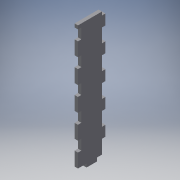
# Autodesk Inventor part: Part2
Saved by Autodesk Inventor 2018 (Build 220112000, 112)
## iProperties
Created: 2018-05-22
Part Number: Part2
Material: Generic
Document SubType Name: Modeling
Designer: Administrator
Density: 1 g/cm^3
Appearance: Default
Author: Administrator
Autodesk Inventor part; units mm, degrees
ref_plane "YZ Plane" through (0, 0, 0) normal (1, 0, 0) x (0, 1, 0)
ref_plane "XZ Plane" through (0, 0, 0) normal (0, 1, 0) x (-1, 0, 0)
ref_plane "XY Plane" through (0, 0, 0) normal (0, 0, 1) x (1, 0, 0)
sketch "Sketch1" plane through (0, 0, 0) normal (1, 0, 0) x (0, 1, 0)
  line L0 (90.5542, 74.5762) -> (-23.7458, 74.5762)
  line L1 (-23.7458, 74.5762) -> (-23.7458, 49.1762)
  line L2 (-23.7458, 49.1762) -> (90.5542, 49.1762)
  line L3 (90.5542, 49.1762) -> (90.5542, 74.5762)
  line L4 (-23.7458, 66.6387) -> (-26.9208, 66.6387)
  line L5 (-26.9208, 66.6387) -> (-26.9208, 57.1137)
  line L6 (-26.9208, 57.1137) -> (-23.7458, 57.1137)
  line L7 (-23.7458, 57.1137) -> (-23.7458, 66.6387)
  point P0 (0, 0)
  dimension "d0" = 25.4
  dimension "d1" = 114.3
  dimension "d4" = 3.175
  dimension "d5" = 7.9375
  dimension "d6" = 7.9375
  constraints: 16 end point, 4 parallel, 2 horizontal, 2 perpendicular, 1 point on line
  measures "d0" distance between parallel lines of L2 L0
  measures "d1" distance between parallel lines of L3 L1
  measures "d4" distance between parallel lines of L1 L5
  measures "d5" distance between parallel lines of L2 L6
  measures "d6" distance between parallel lines of L0 L4
extrude "Extrusion2" add sketch "Sketch1" along normal blind 3.175
sketch "Sketch4" plane through (3.175, 0, 0) normal (1, 0, 0) x (0, 0, -1)
  line L0 (-49.1762, 90.5542) -> (-74.5762, 90.5542) projected
  line L1 (-66.6387, 90.5542) -> (-57.1137, 90.5542)
  line L2 (-57.1137, 90.5542) -> (-57.1137, 87.3792)
  line L3 (-57.1137, 87.3792) -> (-66.6387, 87.3792)
  line L4 (-66.6387, 87.3792) -> (-66.6387, 90.5542)
  line L5 (-49.1762, -23.7458) -> (-49.1762, 90.5542) projected
  line L6 (-74.5762, 90.5542) -> (-74.5762, -23.7458) projected
  line L7 (-74.5762, -11.0458) -> (-71.4012, -11.0458)
  line L8 (-71.4012, -11.0458) -> (-71.4012, -1.5208)
  line L9 (-71.4012, -1.5208) -> (-74.5762, -1.5208)
  line L10 (-74.5762, -1.5208) -> (-74.5762, -11.0458)
  line L11 (-74.5762, -23.7458) -> (-66.6387, -23.7458) projected
  line L12 (-74.5762, 11.1792) -> (-71.4012, 11.1792)
  line L13 (-71.4012, 11.1792) -> (-71.4012, 20.7042)
  line L14 (-71.4012, 20.7042) -> (-74.5762, 20.7042)
  line L15 (-74.5762, 20.7042) -> (-74.5762, 11.1792)
  line L16 (-74.5762, 33.4042) -> (-71.4012, 33.4042)
  line L17 (-71.4012, 33.4042) -> (-71.4012, 42.9292)
  line L18 (-71.4012, 42.9292) -> (-74.5762, 42.9292)
  line L19 (-74.5762, 42.9292) -> (-74.5762, 33.4042)
  line L20 (-71.4012, 55.6292) -> (-74.5762, 55.6292)
  line L21 (-74.5762, 55.6292) -> (-74.5762, 65.1542)
  line L22 (-74.5762, 65.1542) -> (-71.4012, 65.1542)
  line L23 (-71.4012, 65.1542) -> (-71.4012, 55.6292)
  line L24 (-71.4012, 77.8542) -> (-74.5762, 77.8542)
  line L25 (-74.5762, 77.8542) -> (-74.5762, 87.3792)
  line L26 (-74.5762, 87.3792) -> (-71.4012, 87.3792)
  line L27 (-71.4012, 87.3792) -> (-71.4012, 77.8542)
  line L28 (-49.1762, -23.7458) -> (-52.3512, -23.7458)
  line L29 (-52.3512, -23.7458) -> (-52.3512, -11.0458)
  line L30 (-52.3512, -11.0458) -> (-49.1762, -11.0458)
  line L31 (-49.1762, -11.0458) -> (-49.1762, -23.7458)
  line L32 (-49.1762, -1.5208) -> (-52.3512, -1.5208)
  line L33 (-52.3512, -1.5208) -> (-52.3512, 11.1792)
  line L34 (-52.3512, 11.1792) -> (-49.1762, 11.1792)
  line L35 (-49.1762, 11.1792) -> (-49.1762, -1.5208)
  line L36 (-49.1762, 20.7042) -> (-52.3512, 20.7042)
  line L37 (-52.3512, 20.7042) -> (-52.3512, 33.4042)
  line L38 (-52.3512, 33.4042) -> (-49.1762, 33.4042)
  line L39 (-49.1762, 33.4042) -> (-49.1762, 20.7042)
  line L40 (-49.1762, 42.9292) -> (-52.3512, 42.9292)
  line L41 (-52.3512, 42.9292) -> (-52.3512, 55.6292)
  line L42 (-52.3512, 55.6292) -> (-49.1762, 55.6292)
  line L43 (-49.1762, 55.6292) -> (-49.1762, 42.9292)
  line L44 (-49.1762, 65.1542) -> (-52.3512, 65.1542)
  line L45 (-52.3512, 65.1542) -> (-52.3512, 77.8542)
  line L46 (-52.3512, 77.8542) -> (-49.1762, 77.8542)
  line L47 (-49.1762, 77.8542) -> (-49.1762, 65.1542)
  line L48 (-49.1762, 87.3792) -> (-52.3512, 87.3792)
  line L49 (-52.3512, 87.3792) -> (-52.3512, 90.5542)
  line L50 (-52.3512, 90.5542) -> (-49.1762, 90.5542)
  line L51 (-49.1762, 90.5542) -> (-49.1762, 87.3792)
  point P0 (0, 0)
  dimension "d30" = 3.175
  dimension "d31" = 7.9375
  dimension "d32" = 7.9375
  dimension "d33" = 3.175
  dimension "d34" = 9.525
  dimension "d35" = 12.7
  dimension "d36" = 9.525
  dimension "d37" = 12.7
  dimension "d38" = 9.525
  dimension "d39" = 12.7
  dimension "d40" = 9.525
  dimension "d41" = 12.7
  dimension "d42" = 12.7
  dimension "d43" = 9.525
  dimension "d44" = 3.175
  constraints: 96 end point, 24 parallel, 16 point on line, 12 horizontal, 12 perpendicular, 1 midpoint
  measures "d30" distance between parallel lines of L0 L3
  measures "d31" distance between parallel lines of L5 L2
  measures "d32" distance between parallel lines of L6 L4
  measures "d33" distance between parallel lines of L6 L8
  measures "d34" distance between parallel lines of L9 L7
  measures "d35" distance between parallel lines of L11 L7
  measures "d36" distance between parallel lines of L14 L12
  measures "d37" distance between parallel lines of L9 L12
  measures "d38" distance between parallel lines of L18 L16
  measures "d39" distance between parallel lines of L14 L16
  measures "d40" distance between parallel lines of L22 L20
  measures "d41" distance between parallel lines of L18 L20
  measures "d42" distance between parallel lines of L22 L24
  measures "d43" distance between parallel lines of L26 L24
  measures "d44" distance between parallel lines of L5 L29
extrude "Extrusion5" cut sketch "Sketch4" against normal blind 3.175 contours L5 L48 L49 L0 | L5 L28 L29 L30 | L5 L32 L33 L34 | L5 L36 L37 L38 | L5 L40 L41 L42 | L5 L44 L45 L46 | L9 L8 L7 L6 | L14 L13 L12 L6 | L18 L17 L16 L6 | L22 L23 L20 L6 | L26 L27 L24 L6
body "Solid2"
